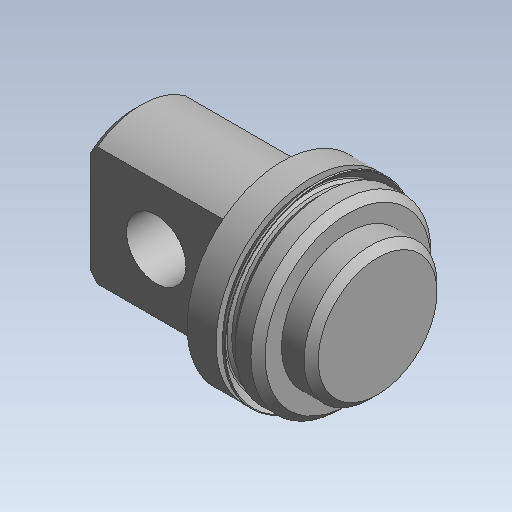
# Autodesk Inventor part: 04PR0K000_rear_head
Saved by Autodesk Inventor 2020 (Build 240168000, 168)
## iProperties
Part Number: 04PR0K000_rear_head
Material: Generic
Catalog Web Link: www.cadenas.de
Description: Rear Head-Original Line - Standard Air Cylinders
Vendor: BIMBA
Document SubType Name: Modeling
Designer: partserver
Manufacturer: BIMBA
Mass: 4.56392 g
Surface Area: 22.1659 cm^2
Volume: 4.56392 cm^3
Density: 1 g/cm^3
Appearance: PSOLRGB-211-211-211
Category: PARTsolutions
Company: BIMBA
PSOL_IDENT_0: {$CADENAS_DATA\23d-libs\bimba\bimba_brand\bimba_imperial\bimba_full_line\original_line_cylinders\sta
PSOL_IDENT_1: ndard_air_cylinders\rear_head.prj},243 {VTYP=3D},{NB=04PR0K000_rear_head},{LINA=04PR0K000_rear_head}
PSOL_IDENT_2: ,{NN=Rear Head},{DATE=19.01.2022 10:19:37},{GEOMDATE=11.01.2022 11:41:00},{VERSION=},{LINEID=40},{WB
PSOL_IDENT_3: VAR=MNT,ACTING,DER,Q,T1,T2,T3,T4,TRIM,Y,K,MB,CUSH,FBON},{WBNUMERIC=TRIM,MB,CUSH}  {NB=04PR0K000_rear
PSOL_IDENT_4: _head},{LINA=04PR0K000_rear_head},{KT=DUMMY},{PN=04PR0K000},{BORE=0.75000},{BOREPN=04},{MNT=P},{MNTA
PSOL_IDENT_5: LG='' , 'Front Nose' , 'P' , 'Rear Pivot' , 'LS' , 'Built-in Valve LS' , 'DX' , 'Double End' , 'BR'
PSOL_IDENT_6: , 'Rear Block' , 'BRT' , 'Rear Trunnion' , 'A' , 'Adjustable Stroke'},{ACTING=R},{ACTINGALG= '' , 'S
PSOL_IDENT_7: ingle Acting' , 'R' , 'Reverse/Double Acting'   },{DER=},{DERALG= '' , 'Standard' },{Q=},{T1=},{T2=}
PSOL_IDENT_8: ,{T3=},{T4=},{TRIM=0},{Y=},{K=K},{KALG= '', 'without K', 'K', 'with K' },{MB=0},{A1=0.2785},{A1N=0.5
PSOL_IDENT_9: 310},{A1P=1.5940},{A1B=1.0940},{A1S=1.2190},{A2=0.156},{A2N=0.2190},{A3=0.0300},{D1=0.8050},{D1N=0.8
PSOL_IDENT_10: 050},{D1P=0.8625},{D1B=0.8325},{D2=0.7615},{C1=0.0300},{C2=0.0000},{NDM=0.4050},{TAB=NPT},{NDMDP=0.3
PSOL_IDENT_11: 020},{D3=0.3440},{A4=0.1880},{A5=0.6200},{D4=0.0000},{A6=0.0000},{A7=0.7500},{A8=0.1250},{D5=0.8170}
PSOL_IDENT_12: ,{D6=0.3120},{A9=0.8440},{NDM2=0.6250},{TAB2=UNF},{C11=0.0300},{C22=0.0000},{C33=0.0227},{C44=0.0300
PSOL_IDENT_13: },{A10=0.3725},{A11=0.0000},{NDM3=0.4050},{NDM3N=0.4050},{NDM3B=0.4050},{TAB3=NPT},{TAB3N=NPT},{TAB3
PSOL_IDENT_14: B=NPT},{A12=0.688},{A12N=0.6880},{A12B=0.6560},{A13=1.3120},{D7=0.2520},{D8=0.6225},{A14=0.0940},{A1
PSOL_IDENT_15: 5=0.0855},{D9=0.5385},{R1=0.0350},{X1=0.0000},{X2=0.0000},{CX=0.0000},{CC=0.0000},{CON=1},{S1=1.0000
PSOL_IDENT_16: },{DB=0.2500},{X1B=0.4380},{X2B=0.0310},{A8B=0.1250},{A9B=0.8750},{MODEL=1},{NDM4=0.1900},{TAB4=UNF}
PSOL_IDENT_17: ,{NDM4DP=0.2500},{BC=1.0000},{B1=0.7150},{B2=0.5000},{B3=0.5000},{ON=1},{ON2=1},{G1=0.1250},{G2=0.56
PSOL_IDENT_18: 20},{G3=0.6250},{G4=0.6250},{GD=0.2520},{G5=0.6250},{G6=0.3725},{RON=0},{H1=1.1175},{H2=0.8170},{H3=
PSOL_IDENT_19: 0.1250},{H4=0.0350},{H5=0.9420},{H6=0.5620},{F=0.4380},{PNUT=1.0000},{CUSH=0},{CC11=0.238},{CC111=0.
PSOL_IDENT_20: 2380},{CC22=0.2750},{CC33=0.1950},{CC44=0.3700},{CC55=0.5350},{CD1=0.1900},{CD2=0.1500},{CD3=0.0725}
PSOL_IDENT_21: ,{CNDM3=0.1380},{CTAB3=UNF},{OLEN=0.6250},{OD=0.3455},{STDIS=0.1560},{STDIS1=0.1560},{BUSHCON=D-3543
PSOL_IDENT_22: },{BUSHL=0.3700},{FBON=0},{LCD=0.0000}
NB: 04PR0K000_rear_head
NN: Rear Head
NT: Original Line - Standard Air Cylinders
NBSYN: $PN._rear_head
LINA: 04PR0K000_rear_head
CATALOG: Bimba Products
PN: 04PR0K000
BORE: 0.75
BOREPN: 04
MNT: Rear Pivot
MNTALG: '' , 'Front Nose' , 'P' , 'Rear Pivot' , 'LS' , 'Built-in Valve LS' , 'DX' , 'Double End' , 'BR' , 'Rear Block' , 'BRT' , 'Rear Trunnion' , 'A' , 'Adjustable Stroke'
ACTING: Reverse/Double Acting
DER: Standard
Q: Without Side Ported Rear Head
T1: without T1
T2: without T2
T3: without T3
T4: without T4
TRIM: 0
Y: without Pivot Bushing
K: with K
MB: 0
A1N: 0.531
A1P: 1.594
A1B: 1.094
A1S: 1.219
A2N: 0.219
A3: 0.03
D1N: 0.805
D1P: 0.8625
D1B: 0.8325
D2: 0.7615
C1: 0.03
C2: 0
TAB: NPT
NDMDP: 0.302
D3: 0.344
A4: 0.188
A5: 0.62
D4: 0
A6: 0
A7: 0.75
A8: 0.125
D5: 0.817
D6: 0.312
A9: 0.844
NDM2: 0.625
TAB2: UNF
C11: 0.03
C22: 0
C33: 0.0227
C44: 0.03
A10: 0.3725
A11: 0
NDM3N: 0.405
NDM3B: 0.405
TAB3N: NPT
TAB3B: NPT
A12N: 0.688
A12B: 0.656
A13: 1.312
D7: 0.252
D8: 0.6225
A14: 0.094
A15: 0.0855
D9: 0.5385
R1: 0.035
X1: 0
X2: 0
CX: 0
CC: 0
S1: 1
DB: 0.25
X1B: 0.438
X2B: 0.031
A8B: 0.125
A9B: 0.875
NDM4: 0.19
TAB4: UNF
NDM4DP: 0.25
BC: 1
B1: 0.715
B2: 0.5
B3: 0.5
G1: 0.125
G2: 0.562
G3: 0.625
G4: 0.625
GD: 0.252
G5: 0.625
G6: 0.3725
H2: 0.817
H3: 0.125
F: 0.438
CUSH: 0
CC111: 0.238
CC22: 0.275
CC33: 0.195
CC44: 0.37
CC55: 0.535
CD1: 0.19
CD2: 0.15
CD3: 0.0725
CNDM3: 0.138
CTAB3: UNF
OD: 0.3455
STDIS1: 0.156
BUSHCON: D-3543
BUSHL: 0.37
FBON: 0
LCD: 0
SUPPLIER: BIMBA
ARTICLENO: 04PR0K000_rear_head
BOMINFO: 04PR0K000_rear_head
CREATOR: CADENAS GmbH
Title: 04PR0K000_rear_head
Author: Cadenas PARTsolutions
Comments: Original Line - Standard Air Cylinders
Autodesk Inventor part; units mm, degrees
sketch "Sketch_1" plane through (0, 0, 0) normal (0, 0, 1) x (1, 0, 0)
  line L0 (7.0739, 0) -> (0, 0)
  line L1 (0, 0) -> (0, 8.9091)
  line L2 (0, 8.9091) -> (0.762, 9.671)
  line L3 (0.762, 9.671) -> (2.4384, 9.671)
  line L4 (2.4384, 9.671) -> (3.2004, 8.9091)
  line L5 (3.2004, 8.9091) -> (3.9624, 8.9091)
  line L6 (3.9624, 8.9091) -> (3.9624, 10.2235)
  line L7 (3.9624, 10.2235) -> (7.0739, 10.2235)
  line L8 (7.0739, 10.2235) -> (7.0739, 0)
  line L9 (7.0739, 0) -> (0, 0)
  constraints: 20 end point
revolve "Revolution1" add sketch "Sketch_1" angle 360 about axis through (7.0739, 0, 0) along (1, 0, 0)
sketch "Sketch_24" plane through (0, 0, 0) normal (0, 0, 1) x (1, 0, 0)
  line L0 (3.9624, 0) -> (3.2004, 0)
  line L1 (3.0477, 10.2235) -> (3.0477, 10.1393)
  line L2 (3.0477, 10.1393) -> (3.8399, 9.3472)
  arc A0 (3.8399, 9.1676) -> (3.8399, 9.3472) centre (3.7501, 9.2574) ccw
  line L3 (3.8399, 9.1676) -> (3.5814, 8.9091)
  line L4 (3.5814, 8.9091) -> (3.2004, 8.9091)
  line L5 (3.2004, 8.9091) -> (3.2004, 8.655)
  line L6 (3.2004, 8.655) -> (3.9624, 8.655)
  line L7 (3.9624, 8.655) -> (3.9624, 9.512)
  line L8 (3.9624, 9.512) -> (3.2509, 10.2235)
  line L9 (3.2509, 10.2235) -> (3.0477, 10.2235)
  constraints: 20 end point, 2 point on circle, 1 centre point
revolve "Revolution2" add sketch "Sketch_24" angle 360 about axis through (3.9624, 0, 0) along (1, 0, 0)
sketch "Sketch_26" plane through (0, 0, 0) normal (0, 0, 1) x (1, 0, 0)
  line L0 (0, 0) -> (-3.175, 0)
  line L1 (-3.175, 0) -> (-3.175, 6.3754)
  line L2 (-3.175, 6.3754) -> (-2.413, 7.1374)
  line L3 (-2.413, 7.1374) -> (0, 7.1374)
  line L4 (0, 7.1374) -> (0, 0)
  line L5 (0, 0) -> (-3.175, 0)
  constraints: 12 end point
revolve "Revolution3" add sketch "Sketch_26" angle 360 about axis through (0, 0, 0) along (1, 0, 0)
sketch "Sketch_27" plane through (0, 0, 0) normal (0, 0, 1) x (1, 0, 0)
  line L0 (22.9489, 0) -> (7.0739, 0)
  line L1 (7.0739, 0) -> (7.0739, 7.9375)
  line L2 (7.0739, 7.9375) -> (22.1869, 7.9375)
  line L3 (22.1869, 7.9375) -> (22.9489, 7.1755)
  line L4 (22.9489, 7.1755) -> (22.9489, 0)
  line L5 (22.9489, 0) -> (7.0739, 0)
  constraints: 12 end point
revolve "Revolution4" add sketch "Sketch_27" angle 360 about axis through (22.9489, 0, 0) along (1, 0, 0)
sketch "Sketch_28" plane through (7.2009, 0, 0) normal (1, 0, 0) x (0, 0, -1)
  line L0 (-15.875, 15.875) -> (-15.875, -15.875)
  line L1 (-15.875, -15.875) -> (15.875, -15.875)
  line L2 (15.875, -15.875) -> (15.875, 15.875)
  line L3 (15.875, 15.875) -> (-15.875, 15.875)
  line L4 (-12.7, 4.7308) -> (-12.7, -4.7308)
  line L5 (-12.7, -4.7308) -> (12.7, -4.7308)
  line L6 (12.7, -4.7308) -> (12.7, 4.7308)
  line L7 (12.7, 4.7308) -> (-12.7, 4.7308)
  constraints: 16 end point
extrude "Extrusion1" cut sketch "Sketch_28" along normal blind 15.875
sketch "Sketch_29" plane through (0, 0, 0) normal (0, 1, 0) x (-1, 0, 0)
  circle A0 centre (-15.875, 0) radius 3.2004
  constraints: 1 centre point
extrude "Extrusion2" cut sketch "Sketch_29" along normal mid plane 18.923
ref_plane "1_XY" through (7.0739, 0, 0) normal (1, 0, 0) x (0, 0, -1)
ref_plane "1_YZ" through (7.0739, 0, 0) normal (0, 0, -1) x (0, 1, 0)
ref_plane "1_ZX" through (7.0739, 0, 0) normal (0, 1, 0) x (1, 0, 0)
ref_plane "lovra_XY" through (7.0739, 0, 0) normal (1, 0, 0) x (0, 1, 0)
ref_plane "lovra_YZ" through (7.0739, 0, 0) normal (0, 1, 0) x (0, 0, 1)
ref_plane "lovra_ZX" through (7.0739, 0, 0) normal (0, 0, 1) x (1, 0, 0)
ref_plane "lovra1_XY" through (2.2987, 0, 0) normal (1, 0, 0) x (0, 0, -1)
ref_plane "lovra1_YZ" through (2.2987, 0, 0) normal (0, 0, -1) x (0, 1, 0)
ref_plane "lovra1_ZX" through (2.2987, 0, 0) normal (0, 1, 0) x (1, 0, 0)
ref_plane "lovra2_XY" through (2.2987, 7.874, 0) normal (1, 0, 0) x (0, 0, -1)
ref_plane "lovra2_YZ" through (2.2987, 7.874, 0) normal (0, 0, -1) x (0, 1, 0)
ref_plane "lovra2_ZX" through (2.2987, 7.874, 0) normal (0, 1, 0) x (1, 0, 0)
ref_plane "lovra21_XY" through (0, 0, 5.2705) normal (1, 0, 0) x (0, 0, -1)
ref_plane "lovra21_YZ" through (0, 0, 5.2705) normal (0, 0, -1) x (0, 1, 0)
ref_plane "lovra21_ZX" through (0, 0, 5.2705) normal (0, 1, 0) x (1, 0, 0)
ref_plane "lovra22_XY" through (0, 0, -5.2705) normal (1, 0, 0) x (0, 0, -1)
ref_plane "lovra22_YZ" through (0, 0, -5.2705) normal (0, 0, -1) x (0, 1, 0)
ref_plane "lovra22_ZX" through (0, 0, -5.2705) normal (0, 1, 0) x (1, 0, 0)
ref_plane "lovra3_XY" through (2.2987, -7.874, 0) normal (1, 0, 0) x (0, 0, -1)
ref_plane "lovra3_YZ" through (2.2987, -7.874, 0) normal (0, 0, -1) x (0, 1, 0)
ref_plane "lovra3_ZX" through (2.2987, -7.874, 0) normal (0, 1, 0) x (1, 0, 0)
ref_plane "olen_XY" through (15.875, 0, 0) normal (1, 0, 0) x (0, 0, -1)
ref_plane "olen_YZ" through (15.875, 0, 0) normal (0, 0, -1) x (0, 1, 0)
ref_plane "olen_ZX" through (15.875, 0, 0) normal (0, 1, 0) x (1, 0, 0)
ref_plane "p1_XY" through (22.9489, 0, 4.7308) normal (1, 0, 0) x (0, 0, -1)
ref_plane "p1_YZ" through (22.9489, 0, 4.7308) normal (0, 0, -1) x (0, 1, 0)
ref_plane "p1_ZX" through (22.9489, 0, 4.7308) normal (0, 1, 0) x (1, 0, 0)
ref_plane "p2_XY" through (22.9489, 0, -4.7308) normal (1, 0, 0) x (0, 0, -1)
ref_plane "p2_YZ" through (22.9489, 0, -4.7308) normal (0, 0, -1) x (0, 1, 0)
ref_plane "p2_ZX" through (22.9489, 0, -4.7308) normal (0, 1, 0) x (1, 0, 0)
ref_plane "port2_XY" through (22.9489, 0, 0) normal (1, 0, 0) x (0, 0, -1)
ref_plane "port2_YZ" through (22.9489, 0, 0) normal (0, 0, -1) x (0, 1, 0)
ref_plane "port2_ZX" through (22.9489, 0, 0) normal (0, 1, 0) x (1, 0, 0)
ref_plane "thd1_XY" through (22.9489, 0, 7.9375) normal (1, 0, 0) x (0, 0, -1)
ref_plane "thd1_YZ" through (22.9489, 0, 7.9375) normal (0, 0, -1) x (0, 1, 0)
ref_plane "thd1_ZX" through (22.9489, 0, 7.9375) normal (0, 1, 0) x (1, 0, 0)
ref_plane "thd2_XY" through (22.9489, 0, -7.9375) normal (1, 0, 0) x (0, 0, -1)
ref_plane "thd2_YZ" through (22.9489, 0, -7.9375) normal (0, 0, -1) x (0, 1, 0)
ref_plane "thd2_ZX" through (22.9489, 0, -7.9375) normal (0, 1, 0) x (1, 0, 0)
ref_plane "to_mounting_bracket_XY" through (23.0124, 0, 0) normal (1, 0, 0) x (0, 0, -1)
ref_plane "to_mounting_bracket_YZ" through (23.0124, 0, 0) normal (0, 0, -1) x (0, 1, 0)
ref_plane "to_mounting_bracket_ZX" through (23.0124, 0, 0) normal (0, 1, 0) x (1, 0, 0)
ref_plane "to_nut_XY" through (25.4, 0, 0) normal (1, 0, 0) x (0, 0, -1)
ref_plane "to_nut_YZ" through (25.4, 0, 0) normal (0, 0, -1) x (0, 1, 0)
ref_plane "to_nut_ZX" through (25.4, 0, 0) normal (0, 1, 0) x (1, 0, 0)
ref_plane "to_pin_XY" through (15.875, 0, 0) normal (0, 1, 0) x (1, 0, 0)
ref_plane "to_pin_YZ" through (15.875, 0, 0) normal (1, 0, 0) x (0, 0, -1)
ref_plane "to_pin_ZX" through (15.875, 0, 0) normal (0, 0, -1) x (0, 1, 0)
ref_plane "to_pin_1_XY" through (15.875, 0, 0) normal (0, 0, 1) x (1, 0, 0)
ref_plane "to_pin_1_YZ" through (15.875, 0, 0) normal (1, 0, 0) x (0, 1, 0)
ref_plane "to_pin_1_ZX" through (15.875, 0, 0) normal (0, 1, 0) x (0, 0, 1)
ref_plane "to_pin_r_XY" through (15.875, 0, 0) normal (0, 0, 1) x (1, 0, 0)
ref_plane "to_pin_r_YZ" through (15.875, 0, 0) normal (1, 0, 0) x (0, 1, 0)
ref_plane "to_pin_r_ZX" through (15.875, 0, 0) normal (0, 1, 0) x (0, 0, 1)
ref_plane "to_screw_XY" through (17.4752, -6.0452, -2.032) normal (0, 0, -1) x (1, 0, 0)
ref_plane "to_screw_YZ" through (17.4752, -6.0452, -2.032) normal (1, 0, 0) x (0, -1, 0)
ref_plane "to_screw_ZX" through (17.4752, -6.0452, -2.032) normal (0, -1, 0) x (0, 0, -1)
ref_plane "to_tube_XY" through (3.2004, 0, 0) normal (1, 0, 0) x (0, 0, -1)
ref_plane "to_tube_YZ" through (3.2004, 0, 0) normal (0, 0, -1) x (0, 1, 0)
ref_plane "to_tube_ZX" through (3.2004, 0, 0) normal (0, 1, 0) x (1, 0, 0)
body "Solid1"
